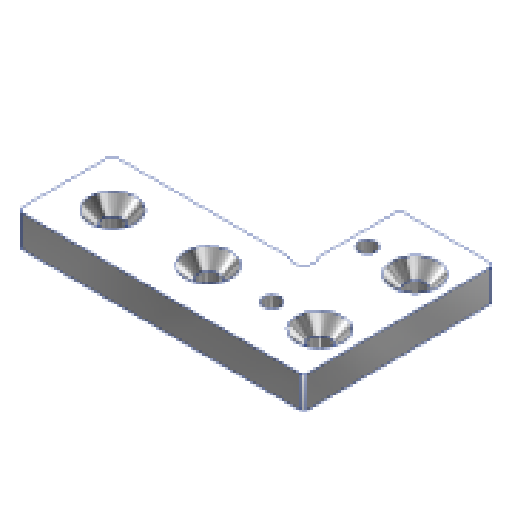
# Autodesk Inventor part: Chapa Suporte 1R (Trilho Roletado)
Saved by Autodesk Inventor 2026.1 (Build 301233000, 233)
## iProperties
Company: Elgin
Created: 2025-09-16
Part Number: Chapa Suporte 1R (Trilho Roletado)
Checked By: Antonio Lucas
Engr Approved By: Antonio Lucas
Material: Aluminio 1060
Document SubType Name: Modeling
Mfg Approved By: Anderson Oliveira
Designer: Willian Pinheiro
Mass: 88.5843 g
Surface Area: 107.907 cm^2
Volume: 32.809 cm^3
Density: 2.7 g/cm^3
Appearance: Alumínio - Plano
Description: Chapa Suporte 1R (Trilho Roletado)
Dimensões: 10 x 60 x 90 mm
Total: 2
Author: Willian Pinheiro
Title: Ceteva
Revision Number: 00
Autodesk Inventor part; units mm, degrees
ref_plane "YZ Plane" through (0, 0, 0) normal (1, 0, 0) x (0, 1, 0)
ref_plane "XZ Plane" through (0, 0, 0) normal (0, 1, 0) x (-1, 0, 0)
ref_plane "XY Plane" through (0, 0, 0) normal (0, 0, 1) x (1, 0, 0)
sketch "Esboço1" plane through (0, 0, 0) normal (0, 0, 1) x (1, 0, 0)
  line L0 (-63.02, 0) -> (63.12, 0) construction
  line L1 (0, -42.02) -> (0, 42.12) construction
  line L2 (-45, 30) -> (45, 30)
  line L3 (45, 30) -> (45, -30)
  line L4 (45, -30) -> (-45, -30)
  line L5 (-45, -30) -> (-45, 30)
  line L6 (-15, 30) -> (45, 30) construction
  line L7 (45, 30) -> (45, 0) construction
  line L8 (45, 0) -> (-15, 0) construction
  line L9 (-15, 0) -> (-15, 30) construction
  line L10 (-15.1, 30.1) -> (45.1, 30.1)
  line L11 (45.1, 30.1) -> (45.1, -0.1)
  line L12 (45.1, -0.1) -> (-15.1, -0.1)
  line L13 (-15.1, -0.1) -> (-15.1, 30.1)
  line L14 (-25, 30) -> (-15, 30) construction
  line L15 (-15, 30) -> (-15, -30) construction
  line L16 (-15, -30) -> (-25, -30) construction
  line L17 (-25, -30) -> (-25, 30) construction
  line L18 (-45, 15) -> (45, 15) construction
  line L19 (-45, -15) -> (45, -15) construction
  line L20 (-20, -30) -> (-20, 30) construction
  line L21 (-35, 30) -> (-35, -30) construction
  line L22 (15, 30) -> (15, -30) construction
  circle A0 centre (-13, 2) radius 3
  point P0 (0, 0)
  point P1 (-20, 15)
  point P2 (-20, -15)
  point P3 (0, -15)
  point P4 (30, -15)
  point P5 (-35, 15)
  point P6 (-35, -15)
  point P7 (45, -0.1)
  point P8 (-15.1, 30)
  point P9 (-10.8576, -0.1)
  point P10 (-15.1, 4.1424)
  dimension "d0" = 60
  dimension "d1" = 90
  dimension "d2" = 60
  dimension "d3" = 30
  dimension "d4" = 0.1
  dimension "d5" = 10
  dimension "d6" = 30
  dimension "d7" = 30
  dimension "d17" = 6
  dimension "d18" = 2
  dimension "d19" = 2
  constraints: 42 end point, 17 point on line, 8 parallel, 8 perpendicular, 6 midpoint, 3 horizontal, 1 centre point, 1 collinear, 1 symmetric about line, 7 other
  measures "d0" distance of L4.end L2.start
  measures "d1" distance of L2.start L2.end
  measures "d2" distance of L7.end L8.end
  measures "d3" distance between parallel lines of L2 L8
  measures "d4" distance between parallel lines of L9 L13
  measures "d5" distance between parallel lines of L17 L15
  measures "d6" distance between parallel lines of L18 L19
  measures "d7" distance of point (30, -15) point (0, -15)
  measures "d17" diameter of A0
  measures "d18" distance from line of A0.centre L15
  measures "d19" distance from line of A0.centre L0
extrude "Extrusão1" add sketch "Esboço1" against normal blind 10 contours L2 L13 A0 L12 L3 L4 L5 | L2 L3 L12 A0 L13 | A0 L12 L13 | L13 L12 A0
extrude "Extrusão2" cut sketch "Esboço1" against normal through all contours L2 L3 L12 A0 L13 | A0 L12 L13 | L13 L12 A0
hole "Furo1" at (0, -15, 0) at (30, -15, 0) at (-35, 15, 0) at (-35, -15, 0) direction (0, 0, -1) diameter 6.5 end through all countersink diameter 14.5 countersink angle 90 clearance for "Countersunk Flat Head Hex Socket Screw ISO 10642" size "M6" standard "ISO"
sketch "Esboço2" plane through (0, 0, -10) normal (0, 0, -1) x (-1, 0, 0)
  point P0 (0, 0)
  point P1 (20, 15)
  point P2 (20, -15)
hole "Furo2" at (-20, 15, -10) at (-20, -15, -10) direction (0, 0, 1) diameter 5.5 end through all countersink diameter 12.5 countersink angle 90 clearance for "Countersunk Flat Head Hex Socket Screw ISO 10642" size "M5" standard "ISO"
chamfer "Chanfro1" distance 1 angle 45 5 edges at (-45, 30, -5) (-15.1, 30, -5) (-45, -30, -5) (45, -30, -5) (45, -0.1, -5)
fillet "Arredondamento1" radius 2 2 edges at (-15.1, 4.1424, -5) (-10.8576, -0.1, -5)
mirror "Espelhar1" about plane through (0, 0, 0) normal (1, 0, 0) remove original yes
equation "\"d18\" = 0.333333 * d17"
equation "\"d19\" = d18"
